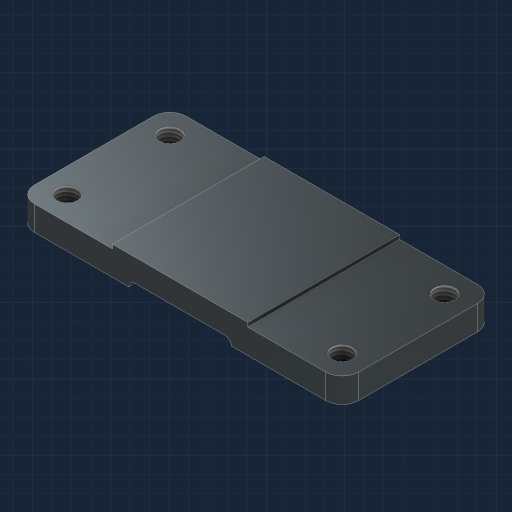
# Autodesk Inventor part: 01-base
Saved by Autodesk Inventor 2024 (Build 280153000, 153)
## iProperties
Created: 2025-03-09
Part Number: 01-base
Material: Iron, Gray
Document SubType Name: Modeling
Designer: DuctopwH
Density: 7.15 g/cm^3
Appearance: Iron Gray
Author: DuctopwH
Autodesk Inventor part; units mm, degrees
ref_plane "YZ Plane" through (0, 0, 0) normal (1, 0, 0) x (0, 1, 0)
ref_plane "XZ Plane" through (0, 0, 0) normal (0, 1, 0) x (-1, 0, 0)
ref_plane "XY Plane" through (0, 0, 0) normal (0, 0, 1) x (1, 0, 0)
sketch "Sketch1" plane through (0, 0, 0) normal (0, 0, 1) x (1, 0, 0)
  line L0 (33, -5.5) -> (-33, -5.5)
  line L1 (-33, -5.5) -> (-33, 5.5)
  line L2 (-33, 5.5) -> (33, 5.5)
  line L3 (33, 5.5) -> (33, -5.5)
  line L4 (33, -5.5) -> (-33, 5.5) construction
  line L5 (-33, -5.5) -> (33, 5.5) construction
  line L6 (-25, 3.5) -> (-79, 3.5)
  line L7 (-79, 3.5) -> (-79, -8.5)
  line L8 (-79, -8.5) -> (-25, -8.5)
  line L9 (-25, -8.5) -> (-25, 3.5)
  line L10 (0, 0) -> (0, 20.8366) construction
  line L11 (25, 3.5) -> (79, 3.5)
  line L12 (79, 3.5) -> (79, -8.5)
  line L13 (79, -8.5) -> (25, -8.5)
  line L14 (25, -8.5) -> (25, 3.5)
  point P0 (-25, -5.5)
  point P1 (25, -5.5)
  point P2 (33, 3.5)
  point P3 (-33, 3.5)
  dimension "d0" = 158
  dimension "d3" = 50
  dimension "d4" = 66
  dimension "d5" = 3
  dimension "d6" = 12
  dimension "d7" = 14
  constraints: 30 end point, 4 parallel, 4 symmetric about line, 2 horizontal, 2 midpoint, 2 perpendicular, 1 vertical
  measures "d0" distance between parallel lines of L12 L7
  measures "d3" distance between parallel lines of L14 L9
  measures "d4" distance of L1.end L2.end
  measures "d5" distance between parallel lines of L8 L0
  measures "d6" distance between parallel lines of L13 L11
  measures "d7" distance between parallel lines of L2 L13
extrude "Extrusion1" add sketch "Sketch1" along normal mid plane 74
fillet "Fillet1" radius 3 2 edges at (25, -5.5, 0) (-25, -5.5, 0)
sketch "Sketch3" plane through (-79, 3.5, 37) normal (0, 1, 0) x (1, 0, 0)
  line L0 (46, 0) -> (0, 0) projected
  line L1 (0, 74) -> (0, 0) projected
  point P0 (79, 37)
  point P1 (12, 12)
  dimension "d11" = 12
  dimension "d12" = 12
  measures "d11" distance from line of L0 point (12, 12)
  measures "d12" distance from line of L1 point (12, 12)
hole "Hole1" at (-67, 3.5, 25) direction (0, -1, 0) diameter 10.106 end through all thread size "M12x1.75" class "6H" standard "ISO Metric profile"
pattern_linear "Rectangular Pattern1" count 2 spacing 50 along (0, 0, -1) count 2 spacing 134 along (1, 0, 0) of "Hole1"
fillet "Fillet2" radius 8 4 edges at (-79, -2.5, 37) (-79, -2.5, -37) (79, -2.5, -37) (79, -2.5, 37)
body "Solid1"
